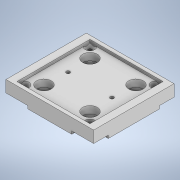
# Autodesk Inventor part: Fuehrungsgrundplatte
Saved by Autodesk Inventor 2022 (Build 260153000, 153)
## iProperties
Created: 2022-04-21
Part Number: Fuehrungsgrundplatte
Material: Generisch
Document SubType Name: Modeling
Designer: 123St
Density: 1 g/cm^3
Appearance: Vorgabe
Author: 123St
Autodesk Inventor part; units mm, degrees
ref_plane "YZ Plane" through (0, 0, 0) normal (1, 0, 0) x (0, 1, 0)
ref_plane "XZ Plane" through (0, 0, 0) normal (0, 1, 0) x (-1, 0, 0)
ref_plane "XY Plane" through (0, 0, 0) normal (0, 0, 1) x (1, 0, 0)
sketch "Skizze1" plane through (0, 0, 0) normal (0, 1, 0) x (-1, 0, 0)
  line L0 (30, -27.5) -> (-30, -27.5)
  line L1 (-30, -27.5) -> (-30, 27.5)
  line L2 (-30, 27.5) -> (30, 27.5)
  line L3 (30, 27.5) -> (30, -27.5)
  line L4 (30, -27.5) -> (-30, 27.5) construction
  line L5 (-30, -27.5) -> (30, 27.5) construction
  point P0 (0, 0)
  dimension "d0" = 60
  dimension "d1" = 55
  constraints: 12 end point, 2 midpoint, 2 parallel, 1 horizontal, 1 perpendicular
  measures "d0" distance of L1.end L2.end
  measures "d1" distance of L0.end L1.end
extrude "Extrusion1" add sketch "Skizze1" along normal blind 10
sketch "Skizze2" plane through (0, 10, 0) normal (0, 1, 0) x (1, 0, 0)
  circle A0 centre (-15.75, 15.75) radius 1.75
  circle A1 centre (15.75, 15.75) radius 1.75
  circle A2 centre (15.75, -15.75) radius 1.75
  circle A3 centre (-15.75, -15.75) radius 1.75
  line L0 (42, 0) -> (-42, 0) projected
  line L1 (0, 38.5) -> (0, -38.5) projected
  point P0 (0, 0)
  dimension "d4" = 31.5
  dimension "d5" = 31.5
  dimension "d6" = 15.75
  dimension "d7" = 31.5
  dimension "d8" = 31.5
  dimension "d9" = 15.75
  dimension "d10" = 15.75
  dimension "d11" = 15.75
  dimension "d12" = 3.5
  dimension "d13" = 3.5
  dimension "d14" = 3.5
  dimension "d15" = 3.5
  constraints: 4 centre point
  measures "d4" distance of A0.centre A1.centre
  measures "d5" distance of A2.centre A1.centre
  measures "d6" distance from line of L0 A2.centre
  measures "d7" distance of A3.centre A2.centre
  measures "d8" distance of A0.centre A3.centre
  measures "d9" distance from line of A2.centre L1
  measures "d10" distance from line of L0 A0.centre
  measures "d11" distance from line of L0 A1.centre
  measures "d12" diameter of A0
  measures "d13" diameter of A1
  measures "d14" diameter of A2
  measures "d15" diameter of A3
extrude "Extrusion2" cut sketch "Skizze2" against normal blind 10
sketch "Skizze3" plane through (0, 10, 0) normal (0, 1, 0) x (1, 0, 0)
  circle A0 centre (-15.75, 15.75) radius 1.75 projected
  circle A1 centre (-15.75, 15.75) radius 5
  circle A2 centre (15.75, 15.75) radius 1.75 projected
  circle A3 centre (15.75, 15.75) radius 5
  circle A4 centre (15.75, -15.75) radius 1.75 projected
  circle A5 centre (15.75, -15.75) radius 5
  circle A6 centre (-15.75, -15.75) radius 1.75 projected
  circle A7 centre (-15.75, -15.75) radius 5
  point P0 (0, 0)
  dimension "d18" = 10
  dimension "d19" = 10
  dimension "d20" = 10
  dimension "d21" = 10
  constraints: 4 centre point, 4 coincident
  measures "d18" diameter of A1
  measures "d19" diameter of A3
  measures "d20" diameter of A7
  measures "d21" diameter of A5
extrude "Extrusion3" cut sketch "Skizze3" against normal blind 7 contours A0 | A1 | A2 | A3 | A4 | A5 | A6 | A7
sketch "Skizze4" plane through (0, 10, 0) normal (0, 1, 0) x (1, 0, 0)
  line L0 (-25, 25) -> (25, 25)
  line L1 (25, 25) -> (25, -25)
  line L2 (25, -25) -> (-25, -25)
  line L3 (-25, -25) -> (-25, 25)
  line L4 (-25, 25) -> (25, -25) construction
  line L5 (25, 25) -> (-25, -25) construction
  point P0 (0, 0)
  dimension "d24" = 50
  dimension "d25" = 50
  constraints: 12 end point, 2 midpoint, 2 parallel, 1 horizontal, 1 perpendicular
  measures "d24" distance of L0.start L0.end
  measures "d25" distance of L2.end L0.start
extrude "Extrusion4" cut sketch "Skizze4" against normal blind 2
sketch "Skizze5" plane through (0, 8, 0) normal (0, 1, 0) x (1, 0, 0)
  circle A0 centre (-15, 0) radius 1.25
  circle A1 centre (15, 0) radius 1.25
  line L0 (0, 38.5) -> (0, -38.5) projected
  line L1 (42, 0) -> (-42, 0) projected
  point P0 (0, 0)
  dimension "d28" = 30
  dimension "d29" = 15
  dimension "d30" = 0
  dimension "d31" = 2.5
  dimension "d32" = 2.5
  constraints: 2 centre point
  measures "d28" distance of A1.centre A0.centre
  measures "d29" distance from line of A1.centre L0
  measures "d30" distance from line of L1 A1.centre
  measures "d31" diameter of A1
  measures "d32" diameter of A0
extrude "Extrusion5" cut sketch "Skizze5" against normal blind 6
sketch "Skizze6" plane through (0, 0, 0) normal (0, 1, 0) x (-1, 0, 0)
  line L0 (37.5, 17.5) -> (-37.5, 17.5)
  line L1 (-37.5, 17.5) -> (-37.5, 22.5)
  line L2 (-37.5, 22.5) -> (-37.5, 22.5)
  line L3 (37.5, 22.5) -> (37.5, 17.5)
  line L4 (37.5, 17.5) -> (-37.5, 22.5) construction
  line L5 (-37.5, 17.5) -> (37.5, 22.5) construction
  line L6 (37.5, -17.5) -> (-37.5, -17.5)
  line L7 (-37.5, -17.5) -> (-37.5, -22.5)
  line L8 (37.5, -22.5) -> (37.5, -17.5)
  line L9 (37.5, -17.5) -> (-37.5, -22.5) construction
  line L10 (-37.5, -17.5) -> (37.5, -22.5) construction
  line L11 (37.5, 22.5) -> (37.5, 32.5)
  line L12 (37.5, 32.5) -> (15, 32.5)
  line L13 (15, 32.5) -> (15, 22.5)
  line L14 (-37.5, 22.5) -> (-37.5, 32.5)
  line L15 (-37.5, 32.5) -> (-15, 32.5)
  line L16 (-15, 32.5) -> (-15, 22.5)
  line L17 (0, -39.5) -> (0, 44.5) projected
  line L18 (37.5, -22.5) -> (37.5, -32.475)
  line L19 (37.5, -32.475) -> (15, -32.475)
  line L20 (15, -32.475) -> (15, -22.475)
  line L21 (-37.5, -22.5) -> (-37.5, -32.475)
  line L22 (-37.5, -32.475) -> (-15, -32.475)
  line L23 (-15, -32.475) -> (-15, -22.475)
  line L24 (-15, 22.5) -> (15, 22.5)
  line L25 (-15, -22.475) -> (15, -22.475)
  line L26 (-37.5, -22.5) -> (-37.5, -22.5)
  line L27 (37.5, -22.5) -> (37.5, -22.5)
  line L28 (37.5, 22.5) -> (37.5, 22.5)
  point P0 (0, 0)
  point P1 (0, 20)
  point P2 (0, -20)
  dimension "d35" = 20
  dimension "d36" = 5
  dimension "d37" = 10
  dimension "d38" = 15
  dimension "d39" = 15
  dimension "d40" = 75
  dimension "d41" = 5
  dimension "d42" = 20
  dimension "d43" = 10
  dimension "d44" = 15
  dimension "d45" = 15
  dimension "d46" = 22.5
  dimension "d47" = 22.5
  dimension "d48" = 22.5
  dimension "d49" = 75
  dimension "d50" = 22.5
  dimension "d51" = 0
  dimension "d52" = 0
  constraints: 56 end point, 11 parallel, 4 horizontal, 4 midpoint, 3 perpendicular, 3 point on line
  measures "d35" distance of point (0, 0) point (0, 20)
  measures "d36" distance of L0.end L1.end
  measures "d37" distance of L15.end L16.end
  measures "d38" distance between parallel lines of L17 L13
  measures "d39" distance between parallel lines of L17 L16
  measures "d40" distance of L0.start L0.end
  measures "d41" distance of L6.end L7.end
  measures "d42" distance of point (0, 0) point (0, -20)
  measures "d43" distance of L22.end L23.end
  measures "d44" distance between parallel lines of L23 L17
  measures "d45" distance between parallel lines of L17 L20
  measures "d46" distance of L14.end L15.end
  measures "d47" distance of L11.end L12.end
  measures "d48" distance of L18.end L19.end
  measures "d49" distance of L6.start L6.end
  measures "d50" distance of L21.end L22.end
  measures "d51" distance between parallel lines of L18 L8
  measures "d52" distance from line of L17 point (0, -20)
extrude "Extrusion6" cut sketch "Skizze6" along normal blind 2
sketch "Skizze7" plane through (0, 2, 0) normal (0, -1, 0) x (1, 0, 0)
  circle A0 centre (-22.5, 22.5) radius 1.25
  circle A1 centre (22.5, 22.5) radius 1.25
  circle A2 centre (22.5, -22.5) radius 1.25
  circle A3 centre (-22.5, -22.5) radius 1.25
  line L0 (0, 38.5) -> (0, -38.5) projected
  line L1 (-42, 0) -> (42, 0) projected
  point P0 (0, 0)
  dimension "d55" = 45
  dimension "d56" = 22.5
  dimension "d57" = 45
  dimension "d58" = 45
  dimension "d59" = 45
  dimension "d60" = 22.5
  dimension "d61" = 22.5
  dimension "d62" = 2.5
  dimension "d63" = 2.5
  dimension "d64" = 2.5
  dimension "d65" = 2.5
  dimension "d71" = 22.5
  constraints: 4 centre point
  measures "d55" distance of A1.centre A0.centre
  measures "d56" distance from line of L0 A0.centre
  measures "d57" distance of A3.centre A0.centre
  measures "d58" distance of A2.centre A3.centre
  measures "d59" distance of A1.centre A2.centre
  measures "d60" distance from line of L1 A0.centre
  measures "d61" distance from line of L1 A1.centre
  measures "d62" diameter of A0
  measures "d63" diameter of A1
  measures "d64" diameter of A2
  measures "d65" diameter of A3
  measures "d71" distance from line of L0 A3.centre
extrude "Extrusion7" cut sketch "Skizze7" against normal blind 6
chamfer "Fase1" distance 2 angle 45 4 edges at (21.25, 8, -22.5) (21.25, 8, 22.5) (-23.75, 8, 22.5) (-23.75, 8, -22.5)
equation "\"d6\" = 0.5 * d5"
equation "\"d9\" = 0.5 * d7"
equation "\"d10\" = 0.5 * d8"
equation "\"d11\" = 0.5 * d5"
equation "\"d29\" = 0.5 * d28"
equation "\"d56\" = 0.5 * d55"
equation "\"d60\" = 0.5 * d57"
equation "\"d61\" = 0.5 * d59"
equation "\"d71\" = 0.5 * d58"
